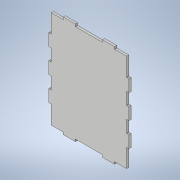
# Autodesk Inventor part: bottom-case
Saved by Autodesk Inventor 2020 (Build 240168000, 168)
## iProperties
Created: 2019-12-17
Part Number: bottom-case
Material: Generic
Document SubType Name: Modeling
Designer: fabfarm
Density: 1 g/cm^3
Appearance: Default
Author: fabfarm
Autodesk Inventor part; units mm, degrees
ref_plane "YZ Plane" through (0, 0, 0) normal (1, 0, 0) x (0, 1, 0)
ref_plane "XZ Plane" through (0, 0, 0) normal (0, 1, 0) x (-1, 0, 0)
ref_plane "XY Plane" through (0, 0, 0) normal (0, 0, 1) x (1, 0, 0)
sketch "Sketch1" plane through (0, 0, 0) normal (0, 0, 1) x (1, 0, 0)
  line L0 (330, -401.45) -> (-330, -401.45)
  line L1 (-330, -401.45) -> (-330, 401.45)
  line L2 (-330, 401.45) -> (330, 401.45)
  line L3 (330, 401.45) -> (330, -401.45)
  line L4 (330, -401.45) -> (-330, 401.45) construction
  line L5 (-330, -401.45) -> (330, 401.45) construction
  point P0 (0, 0)
  dimension "d0" = 802.9
  dimension "d1" = 660
  constraints: 12 end point, 2 midpoint, 2 parallel, 1 horizontal, 1 perpendicular
  measures "d0" distance of L2.end L0.start
  measures "d1" distance of L0.start L0.end
extrude "Extrusion1" add sketch "Sketch1" along normal blind 18.55
sketch "Sketch2" plane through (0, 0, 18.55) normal (0, 0, 1) x (1, 0, 0)
  line L0 (-330, 401.45) -> (-330, -401.45) construction
  line L1 (330, 401.45) -> (-330, 401.45) construction
  line L2 (-330, 401.45) -> (-311.45, 401.45)
  line L3 (-311.45, 401.45) -> (-311.45, 250)
  line L4 (-311.45, 250) -> (-330, 250)
  line L5 (-330, 250) -> (-330, 401.45)
  line L6 (-330, -401.45) -> (330, -401.45) projected
  line L7 (-330, -401.45) -> (-311.45, -401.45)
  line L8 (-311.45, -401.45) -> (-311.45, -250)
  line L9 (-311.45, -250) -> (-330, -250)
  line L10 (-330, -250) -> (-330, -401.45)
  line L11 (-330, -150) -> (-311.45, -150)
  line L12 (-311.45, -150) -> (-311.45, -50)
  line L13 (-311.45, -50) -> (-330, -50)
  line L14 (-330, -50) -> (-330, -150)
  line L15 (-330, 50) -> (-311.45, 50)
  line L16 (-311.45, 50) -> (-311.45, 150)
  line L17 (-311.45, 150) -> (-330, 150)
  line L18 (-330, 150) -> (-330, 50)
  point P0 (0, 0)
  dimension "d21" = 100
  dimension "d22" = 100
  dimension "d23" = 100
  dimension "d24" = 100
  dimension "d26" = 18.55
  dimension "d60" = 100
  constraints: 32 end point, 8 parallel, 5 point on line, 4 horizontal, 4 perpendicular, 3 collinear
  measures "d21" distance between parallel lines of L4 L17
  measures "d22" distance of L15.end L16.end
  measures "d23" distance between parallel lines of L13 L15
  measures "d24" distance of L11.end L12.end
  measures "d26" distance of L0.end L7.end
  measures "d60" distance between parallel lines of L9 L11
extrude "Extrusion2" cut sketch "Sketch2" against normal blind 18.55
mirror "Mirror1" about plane through (0, 0, 0) normal (1, 0, 0) of "Extrusion2"
sketch "Esquisse5" plane through (0, 0, 18.55) normal (0, 0, 1) x (1, 0, 0)
  line L0 (311.45, 401.45) -> (-311.45, 401.45) projected
  line L1 (0, 401.45) -> (0, -401.45) construction
  line L2 (-311.45, -401.45) -> (311.45, -401.45) projected
  line L3 (-330, 250) -> (-311.45, 250) projected
  circle A0 centre (-313.041, 251.591) radius 2.25
  circle A1 centre (-313.041, 148.409) radius 2.25
  line L4 (-330, 50) -> (-311.45, 50) projected
  circle A2 centre (-313.041, 51.591) radius 2.25
  line L5 (-311.45, -150) -> (-311.45, -50) projected
  circle A3 centre (-313.041, -51.591) radius 2.25
  circle A4 centre (-313.041, -148.409) radius 2.25
  line L6 (-311.45, -401.45) -> (-311.45, -250) projected
  circle A5 centre (-313.041, -251.591) radius 2.25
  line L7 (-313.041, 251.591) -> (-311.45, 250) construction
  line L8 (-311.45, 401.45) -> (-311.45, 250) projected
  circle A6 centre (313.041, 251.591) radius 2.25
  circle A7 centre (313.041, 148.409) radius 2.25
  line L9 (330, 50) -> (311.45, 50)
  circle A8 centre (313.041, 51.591) radius 2.25
  circle A9 centre (313.041, -51.591) radius 2.25
  circle A10 centre (313.041, -148.409) radius 2.25
  circle A11 centre (313.041, -251.591) radius 2.25
  line L10 (313.041, 251.591) -> (311.45, 250) construction
  point P0 (0, 0)
  point P1 (-311.45, 150)
  point P2 (311.45, 150)
  point P3 (311.45, -250)
  dimension "d58" = 4.5
  dimension "d59" = 45
  constraints: 11 symmetric about line, 8 end point, 5 vertical alignment, 4 vertical, 2 centre point, 2 midpoint, 32 other
  measures "d59" angle of L8 L7
extrude "Extrusion5" cut sketch "Esquisse5" against normal blind 18.55
sketch "Esquisse7" plane through (0, 0, 18.55) normal (0, 0, 1) x (1, 0, 0)
  line L0 (-311.45, -401.45) -> (311.45, -401.45) projected
  line L1 (-211.45, -401.45) -> (-111.45, -401.45)
  line L2 (-111.45, -401.45) -> (-111.45, -420)
  line L3 (-111.45, -420) -> (-211.45, -420)
  line L4 (-211.45, -420) -> (-211.45, -401.45)
  line L5 (111.45, -401.45) -> (211.45, -401.45)
  line L6 (211.45, -401.45) -> (211.45, -420)
  line L7 (211.45, -420) -> (111.45, -420)
  line L8 (111.45, -420) -> (111.45, -401.45)
  line L9 (-311.45, -250) -> (-311.45, -401.45) projected
  line L10 (311.45, -401.45) -> (311.45, -250) projected
  line L11 (-330, 50) -> (-330, -50) projected
  line L12 (-330, 0) -> (330, 0) construction
  line L13 (330, -50) -> (330, 50) projected
  line L14 (-211.45, 401.45) -> (-111.45, 401.45)
  line L15 (-111.45, 401.45) -> (-111.45, 420)
  line L16 (-111.45, 420) -> (-211.45, 420)
  line L17 (-211.45, 420) -> (-211.45, 401.45)
  line L18 (111.45, 401.45) -> (211.45, 401.45)
  line L19 (211.45, 401.45) -> (211.45, 420)
  line L20 (211.45, 420) -> (111.45, 420)
  line L21 (111.45, 420) -> (111.45, 401.45)
  circle A0 centre (-181.45, -410.725) radius 2.25 construction
  circle A1 centre (-141.45, -410.725) radius 2.25 construction
  circle A2 centre (141.45, -410.725) radius 2.25 construction
  circle A3 centre (181.45, -410.725) radius 2.25 construction
  circle A4 centre (-181.45, 410.725) radius 2.25 construction
  circle A5 centre (-141.45, 410.725) radius 2.25 construction
  circle A6 centre (141.45, 410.725) radius 2.25 construction
  circle A7 centre (181.45, 410.725) radius 2.25 construction
  line L22 (-211.45, -410.725) -> (-111.45, -410.725) construction
  point P0 (0, 0)
  point P1 (-311.45, -251.44)
  point P2 (311.45, -251.44)
  point P3 (-111.45, -401.45)
  dimension "d41" = 100
  dimension "d42" = 100
  dimension "d43" = 100
  dimension "d44" = 100
  dimension "d45" = 18.55
  dimension "d46" = 4.5
  dimension "d47" = 30
  dimension "d48" = 30
  dimension "d49" = 30
  dimension "d50" = 30
  constraints: 36 end point, 12 symmetric about line, 8 centre point, 8 point on line, 4 midpoint, 4 parallel, 3 equal radius, 2 horizontal, 2 perpendicular, 4 other
  measures "d41" distance of L2.end L3.end
  measures "d42" distance of L6.end L7.end
  measures "d43" distance between parallel lines of L9 L4
  measures "d44" distance between parallel lines of L6 L10
  measures "d45" distance of L1.end L2.end
  measures "d46" diameter of A0
  measures "d47" distance from line of L4 A0.centre
  measures "d48" distance from line of L2 A1.centre
  measures "d49" distance from line of L8 A2.centre
  measures "d50" distance from line of L6 A3.centre
extrude "Extrusion7" add sketch "Esquisse7" against normal blind 18.55
sketch "Esquisse8" plane through (0, 0, 18.55) normal (0, 0, 1) x (1, 0, 0)
  line L0 (-211.45, 401.45) -> (-311.45, 401.45) construction
  line L1 (-311.45, -401.45) -> (-211.45, -401.45) projected
  circle A0 centre (-212.5814, -402.5814) radius 1.6
  circle A1 centre (-110.3186, -402.5814) radius 1.6
  line L2 (-111.45, -401.45) -> (111.45, -401.45) projected
  circle A2 centre (110.3186, -402.5814) radius 1.6
  circle A3 centre (212.5814, -402.5814) radius 1.6
  line L3 (212.5814, -402.5814) -> (211.45, -401.45) construction
  line L4 (211.45, -401.45) -> (311.45, -401.45) projected
  line L5 (-330, 50) -> (-330, -50) projected
  line L6 (-330, 0) -> (330, 0) construction
  line L7 (330, -50) -> (330, 50) projected
  circle A4 centre (-212.5814, 402.5814) radius 1.6
  circle A5 centre (-110.3186, 402.5814) radius 1.6
  line L8 (-111.45, 401.45) -> (111.45, 401.45)
  circle A6 centre (110.3186, 402.5814) radius 1.6
  circle A7 centre (212.5814, 402.5814) radius 1.6
  line L9 (212.5814, 402.5814) -> (211.45, 401.45) construction
  point P0 (0, 0)
  point P1 (-111.45, 401.45)
  dimension "d56" = 3.2
  dimension "d57" = 45
  constraints: 8 end point, 8 symmetric about line, 4 horizontal, 3 horizontal alignment, 2 midpoint, 24 other
  measures "d57" angle of L4 L3
extrude "Extrusion8" cut sketch "Esquisse8" against normal blind 18.55
body "Solid1"
